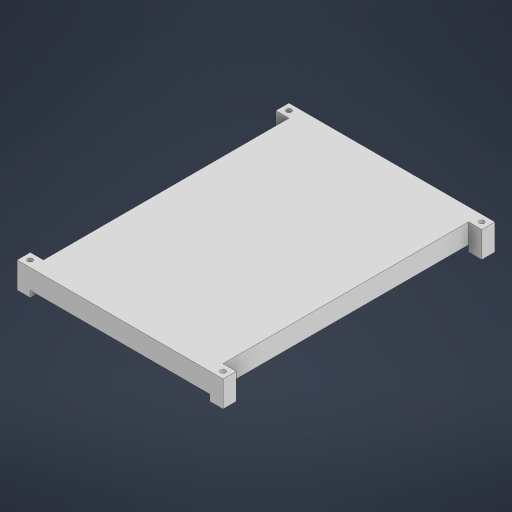
# Autodesk Inventor part: 7InchScreen
Saved by Autodesk Inventor 2023 (Build 270158000, 158)
## iProperties
Created: 2023-02-22
Part Number: 7InchScreen
Material: Generic
Document SubType Name: Modeling
Designer: uzair
Density: 1 g/cm^3
Appearance: Default
Author: uzair
Autodesk Inventor part; units mm, degrees
ref_plane "YZ Plane" through (0, 0, 0) normal (1, 0, 0) x (0, 1, 0)
ref_plane "XZ Plane" through (0, 0, 0) normal (0, 1, 0) x (-1, 0, 0)
ref_plane "XY Plane" through (0, 0, 0) normal (0, 0, 1) x (1, 0, 0)
sketch "Sketch1" plane through (0, 0, 0) normal (0, 1, 0) x (-1, 0, 0)
  line L0 (0, 0) -> (-125, 0)
  line L1 (-125, 0) -> (-125, -165)
  line L2 (-125, -165) -> (0, -165)
  line L3 (0, -165) -> (0, 0)
  circle A0 centre (-4, -4) radius 1.5
  circle A1 centre (-4, -161) radius 1.5
  circle A2 centre (-121, -4) radius 1.5
  circle A3 centre (-121, -161) radius 1.5
  line L4 (-125, 0) -> (-117, 0)
  line L5 (-117, 0) -> (-117, -8)
  line L6 (-117, -8) -> (-125, -8)
  line L7 (-125, -8) -> (-125, 0)
  line L8 (-125, -165) -> (-117, -165)
  line L9 (-117, -165) -> (-117, -157)
  line L10 (-117, -157) -> (-125, -157)
  line L11 (-125, -157) -> (-125, -165)
  line L12 (0, 0) -> (-8, 0)
  line L13 (-8, 0) -> (-8, -8)
  line L14 (-8, -8) -> (0, -8)
  line L15 (0, -8) -> (0, 0)
  line L16 (0, -165) -> (-8, -165)
  line L17 (-8, -165) -> (-8, -157)
  line L18 (-8, -157) -> (0, -157)
  line L19 (0, -157) -> (0, -165)
  line L20 (-117, -8) -> (-125, -8)
  line L21 (-125, -8) -> (-125, -157)
  line L22 (-125, -157) -> (-117, -157)
  line L23 (-117, -157) -> (-117, -8)
  line L24 (0, -8) -> (-8, -8)
  line L25 (-8, -8) -> (-8, -157)
  line L26 (-8, -157) -> (0, -157)
  line L27 (0, -157) -> (0, -8)
  dimension "d0" = 125
  dimension "d1" = 165
  dimension "d2" = 3
  dimension "d3" = 3
  dimension "d4" = 3
  dimension "d5" = 3
  dimension "d8" = 8
  dimension "d9" = 8
  dimension "d10" = 8
  dimension "d11" = 8
  dimension "d12" = 8
  dimension "d13" = 8
  dimension "d14" = 8
  dimension "d15" = 8
  constraints: 56 end point, 14 parallel, 7 horizontal, 7 perpendicular, 4 centre point, 4 coincident
  measures "d0" distance of L2.end L1.end
  measures "d1" distance of L1.end L0.end
  measures "d2" diameter of A0
  measures "d3" diameter of A1
  measures "d4" diameter of A2
  measures "d5" diameter of A3
  measures "d8" distance of L5.end L6.end
  measures "d9" distance of L4.end L5.end
  measures "d10" distance of L10.end L9.end
  measures "d11" distance of L9.end L8.end
  measures "d12" distance of L14.end L13.end
  measures "d13" distance of L13.end L12.end
  measures "d14" distance of L17.end L18.end
  measures "d15" distance of L16.end L17.end
extrude "Extrusion1" add sketch "Sketch1" along normal blind 15.8 contours L3 L14 L13 L0 | L13 L25 L17 L2 L9 L23 L5 L0 | L5 L6 L1 L0 | L3 L2 L17 L18 | L9 L2 L1 L10
sketch "Sketch2" plane through (125, 0, -165) normal (0, 0, -1) x (-1, 0, 0)
  line L0 (8, 15.8) -> (0, 15.8) projected
  line L1 (8, 15.8) -> (117, 15.8)
  line L2 (117, 15.8) -> (117, 0.8)
  line L3 (117, 0.8) -> (8, 0.8)
  line L4 (8, 0.8) -> (8, 15.8)
  line L5 (0, 0) -> (125, 0) projected
  line L6 (8, 0.8) -> (117, 0.8)
  line L7 (117, 0.8) -> (117, 0)
  line L8 (117, 0) -> (8, 0)
  line L9 (8, 0) -> (8, 0.8)
  line L10 (8, 0.8) -> (68, 0.8)
  line L11 (68, 0.8) -> (68, 0)
  line L12 (68, 0) -> (8, 0)
  line L13 (8, 0) -> (8, 0.8)
  dimension "d16" = 109
  dimension "d17" = 15
  dimension "d18" = 60
  dimension "d19" = 0.8
  constraints: 24 end point, 6 parallel, 3 horizontal, 3 perpendicular, 2 point on line
  measures "d16" distance of L2.end L3.end
  measures "d17" distance of L1.end L2.end
  measures "d18" distance of L11.end L12.end
  measures "d19" distance of L10.end L11.end
extrude "Extrusion2" cut sketch "Sketch2" against normal blind 15 contours L3 L11 L5 L9
sketch "Sketch3" plane through (0, 0, 0) normal (0, -1, 0) x (1, 0, 0)
  line L0 (57, -150) -> (117, -150) projected
  line L1 (0, 0) -> (125, 0) projected
  line L2 (117, -150) -> (57, -150)
  line L3 (57, -150) -> (57, 0)
  line L4 (57, 0) -> (117, 0)
  line L5 (117, 0) -> (117, -150)
  line L6 (125, -165) -> (0, -165) projected
  line L7 (57, 0) -> (8, 0)
  line L8 (8, 0) -> (8, -165)
  line L9 (8, -165) -> (57, -165)
  line L10 (57, -165) -> (57, 0)
  line L11 (125, -165) -> (117, -165) projected
  line L12 (117, -165) -> (99.5, -165)
  line L13 (99.5, -165) -> (99.5, -150)
  line L14 (99.5, -150) -> (117, -150)
  line L15 (117, -150) -> (117, -165)
  dimension "d22" = 60
  dimension "d23" = 49
  dimension "d24" = 17.5
  constraints: 24 end point, 6 parallel, 3 horizontal, 3 perpendicular, 3 point on line
  measures "d22" distance of L3.end L4.end
  measures "d23" distance of L9.end L8.end
  measures "d24" distance of L13.end L14.end
extrude "Extrusion3" cut sketch "Sketch3" against normal blind 3.8 contours L3 L1 L5 L0 | L10 L6 L8 L1 L3 | L0 L15 L6 L13
body "Solid1"
